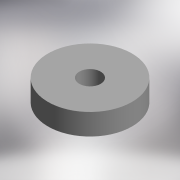
# Autodesk Inventor part: z-linear-encoder-strip-standoff
Saved by Autodesk Inventor 2016 (Build 200138000, 138)
## iProperties
Created: 2015-05-21
Part Number: z-linear-encoder-strip-standoff
Material: Nylon 6/6
Document SubType Name: Modeling
Designer: as
Mass: 0.207355 g
Surface Area: 2.16157 cm^2
Volume: 0.1835 cm^3
Density: 1.13 g/cm^3
Appearance: Nylon 6
Author: as
Autodesk Inventor part; units mm, degrees
ref_plane "YZ Plane" through (0, 0, 0) normal (1, 0, 0) x (0, 1, 0)
ref_plane "XZ Plane" through (0, 0, 0) normal (0, 1, 0) x (-1, 0, 0)
ref_plane "XY Plane" through (0, 0, 0) normal (0, 0, 1) x (1, 0, 0)
sketch "Sketch1" plane through (0, 0, 0) normal (0, 0, 1) x (1, 0, 0)
  circle A0 centre (-53, 0) radius 3.95
  circle A1 centre (-53, 0) radius 1
  point P0 (0, 0)
  dimension "d0" = 7.9
  dimension "d1" = 2
  constraints: 2 centre point, 1 coincident
  measures "d0" diameter of A0
  measures "d1" diameter of A1
extrude "Extrusion1" add sketch "Sketch1" along normal blind 4
body "Solid1"
